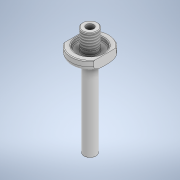
# Autodesk Inventor part: Cartridge Interface Tube
Saved by Autodesk Inventor 2021 (Build 250183000, 183)
## iProperties
Created: 2020-04-22
Part Number: Cartridge Interface Tube
Material: Generic
Document SubType Name: Modeling
Designer: jgray
Density: 1 g/cm^3
Appearance: Default
Author: jgray
Autodesk Inventor part; units mm, degrees
ref_plane "YZ Plane" through (0, 0, 0) normal (1, 0, 0) x (0, 1, 0)
ref_plane "XZ Plane" through (0, 0, 0) normal (0, 1, 0) x (-1, 0, 0)
ref_plane "XY Plane" through (0, 0, 0) normal (0, 0, 1) x (1, 0, 0)
sketch "Sketch1" plane through (0, 0, 0) normal (0, 1, 0) x (-1, 0, 0)
  circle A0 centre (0, 0) radius 6.25
  dimension "d0" = 12.5
  constraints: 1 centre point, 1 coincident
  measures "d0" diameter of A0
extrude "Extrusion1" add sketch "Sketch1" along normal blind 3.2
sketch "Sketch2" plane through (0, 3.2, 0) normal (0, 1, 0) x (1, 0, 0)
  circle A0 centre (0, 0) radius 2.315
  circle A1 centre (0, 0) radius 4.45
  dimension "d3" = 4.63
  dimension "d4" = 8.9
  constraints: 2 centre point, 2 coincident
  measures "d3" diameter of A0
  measures "d4" diameter of A1
extrude "Extrusion2" cut sketch "Sketch2" against normal blind 1.32
fillet "Fillet1" radius 0.25 4 edges at (-4.45, 1.88, 0) (-2.315, 1.88, 0) (-4.45, 3.2, 0) (6.25, 3.2, 0)
fillet "Fillet6" radius 1.5 1 edges at (6.25, 0, 0)
sketch "Sketch3" plane through (0, 3.2, 0) normal (0, 1, 0) x (1, 0, 0)
  circle A0 centre (0, 0) radius 2.5
  dimension "d8" = 5
  constraints: 1 centre point, 1 coincident
  measures "d8" diameter of A0
extrude "Extrusion3" add sketch "Sketch3" along normal blind 5.3
chamfer "Chamfer2" distance 0.2 angle 45 1 edges at (-2.5, 8.5, 0)
chamfer "Chamfer3" distance 0.15 angle 45 1 edges at (-2.5, 3.2, 0)
sketch "Sketch4" plane through (0, 0, 0) normal (0, -1, 0) x (1, 0, 0)
  circle A0 centre (0, 0) radius 6 projected
  circle A1 centre (0, 0) radius 2
  dimension "d20" = 4
  constraints: 1 centre point, 1 coincident
  measures "d20" diameter of A1
extrude "Extrusion4" add sketch "Sketch4" along normal blind 27.5 contours A1
sketch "Sketch5" plane through (0, -27.5, 0) normal (0, -1, 0) x (1, 0, 0)
  circle A0 centre (0, 0) radius 2 projected
  circle A1 centre (0, 0) radius 1.25
  dimension "d23" = 2.5
  constraints: 1 centre point, 1 coincident
  measures "d23" diameter of A1
extrude "Extrusion5" cut sketch "Sketch5" against normal through all contours A1
thread "Thread1" size "M5x0.8" class "6g" standard "ANSI Metric M Profile" full length
fillet "Fillet2" radius 0.219 1 edges at (-1.25, -27.5, 0)
fillet "Fillet3" radius 0.248 1 edges at (-2, -27.5, 0)
sketch "Sketch6" plane through (0, 3.2, 0) normal (0, 1, 0) x (1, 0, 0)
  circle A0 centre (0, 0) radius 6.25 projected
  circle A1 centre (0, 0) radius 6.25
  line L0 (5, 6.4624) -> (-5, 6.4624)
  line L1 (-5, 6.4624) -> (-5, -6.4624)
  line L2 (-5, -6.4624) -> (5, -6.4624)
  line L3 (5, -6.4624) -> (5, 6.4624)
  line L4 (5, 6.4624) -> (-5, -6.4624) construction
  line L5 (-5, 6.4624) -> (5, -6.4624) construction
  point P0 (5, 3.75)
  point P1 (5, -3.75)
  point P2 (-5, -3.75)
  point P3 (-5, 3.75)
  dimension "d30" = 10
  constraints: 12 end point, 2 midpoint, 2 parallel, 1 centre point, 1 coincident, 1 concentric, 1 horizontal, 1 perpendicular
  measures "d30" distance of L2.end L1.end
extrude "Extrusion6" cut sketch "Sketch6" against normal blind 10 contours A0 L3 | L1 A0
fillet "Fillet5" radius 0.25 1 edges at (-2, 0, 0)
body "Solid1"
